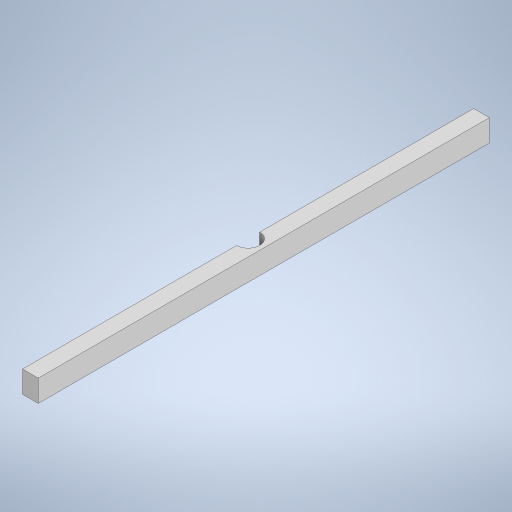
# Autodesk Inventor part: block spacer - v1
Saved by Autodesk Inventor 2023 (Build 270158000, 158)
## iProperties
Created: 2022-07-13
Part Number: block spacer - v1
Material: Generic
Document SubType Name: Modeling
Designer: Caleb
Density: 1 g/cm^3
Appearance: Default
Author: Caleb
Autodesk Inventor part; units mm, degrees
ref_plane "YZ Plane" through (0, 0, 0) normal (1, 0, 0) x (0, 1, 0)
ref_plane "XZ Plane" through (0, 0, 0) normal (0, 1, 0) x (-1, 0, 0)
ref_plane "XY Plane" through (0, 0, 0) normal (0, 0, 1) x (1, 0, 0)
sketch "Sketch1" plane through (0, 0, 0) normal (0, 1, 0) x (-1, 0, 0)
  line L0 (-0.75, 21.55) -> (0.75, 21.55)
  line L1 (0.75, -21.55) -> (-0.75, -21.55)
  line L2 (-0.75, -21.55) -> (-0.75, 21.55)
  line L3 (-0.75, 21.55) -> (0.75, -21.55) construction
  line L4 (0.75, 21.55) -> (-0.75, -21.55) construction
  arc A0 (0.75, 1.1) -> (0.75, -1.1) centre (0.75, 0) ccw
  line L5 (0.75, 21.55) -> (0.75, 1.1)
  line L6 (0.75, -1.1) -> (0.75, -21.55)
  point P0 (0, 0)
  dimension "d0" = 43.1
  dimension "d1" = 1.5
  dimension "d2" = 1.1
  constraints: 14 end point, 4 vertical alignment, 2 equal length, 2 midpoint, 2 point on circle, 1 centre point, 1 horizontal, 1 horizontal alignment, 1 vertical
  measures "d0" distance of L0.end L1.start
  measures "d1" distance of L0.start L0.end
  measures "d2" radius of A0
extrude "Extrusion1" add sketch "Sketch1" along normal blind 2.1
body "Solid1"
